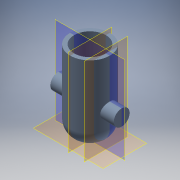
# Autodesk Inventor part: Waterkanon
Saved by Autodesk Inventor 2018 (Build 220112000, 112)
## iProperties
Manager: Pierloot J.
Company: Emmaüs Bovenbouw Aalter
Created: 2015-08-18
Part Number: Waterkanon
Material: S235
Catalog Web Link: http://emmausbovenbouw.op-weg.be/
Vendor: Emmaüsinstituut Bovenbouw Aalter
Document SubType Name: Modeling
Designer: Pierlootj
Engineer: Pierloot J.
Manufacturer: Standard
Standards Organization: Custom
Density: 7.86 g/cm^3
Appearance: Light Steel Blue
Title: Algemene titel
Subject: Specifieke titel
Author: Pierlootj
Keywords: Ruwe Ø xxxxx
Comments: Opmerking
Autodesk Inventor part; units mm, degrees
sketch "Sketch19" plane through (0, 0, 0) normal (0, 0, 1) x (1, 0, 0)
  circle A0 centre (0, 0) radius 12.5
  dimension "d130" = 25
  constraints: 1 centre point, 1 coincident
  measures "d130" diameter of A0
extrude "Extrusion17" add sketch "Sketch19" along normal blind 50
sketch "Sketch20" plane through (0, 0, 50) normal (0, 0, 1) x (1, 0, 0)
  circle A0 centre (0, 0) radius 10
  dimension "d133" = 20
  constraints: 1 centre point, 1 coincident
  measures "d133" diameter of A0
fillet "Fillet6" radius 10 1 edges at (-12.5, 0, 0)
extrude "Extrusion18" cut sketch "Sketch20" against normal blind 40
ref_plane "Work Plane3" through (10, 0, 0) normal (1, 0, 0) x (0, 1, 0)
sketch "Sketch21" plane through (10, 0, 0) normal (1, 0, 0) x (0, 1, 0)
  line L0 (0, 0) -> (0, 20)
  circle A0 centre (0, 20) radius 5
  dimension "d138" = 20
  dimension "d139" = 10
  constraints: 2 end point, 1 centre point, 1 coincident, 1 vertical
  measures "d138" distance of L0.start L0.end
  measures "d139" diameter of A0
extrude "Extrusion19" add sketch "Sketch21" along normal blind 10
mirror "Mirror1" about plane through (0, 0, 0) normal (1, 0, 0) of "Extrusion19"
sketch "Sketch22" plane through (-20, 0, 20) normal (-1, 0, 0) x (0, 0, 1)
  circle A0 centre (0, 0) radius 2.5
  point P0 (-20, 0)
  dimension "d142" = 5
  constraints: 1 centre point
  measures "d142" diameter of A0
extrude "Extrusion20" cut sketch "Sketch22" against normal blind 3
body "Solid8"
